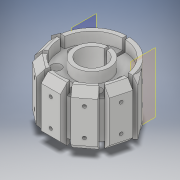
# Autodesk Inventor part: Sensor_Mount
Saved by Autodesk Inventor 2019.3 (Build 233278000, 278)
## iProperties
Created: 2019-04-10
Part Number: Sensor_Mount
Material: Типовые
Document SubType Name: Modeling
Designer: Andrew
Density: 1 g/cm^3
Appearance: По умолчанию
Author: Andrew
## iProperties of the stored document Sensor_Mount_3DПЕЧАТЬ.ipt
Created: 2019-04-10
Part Number: Sensor_Mount_3DПЕЧАТЬ
Material: Типовые
Document SubType Name: Modeling
Designer: Andrew
Density: 1 g/cm^3
Appearance: По умолчанию
Author: Andrew
Autodesk Inventor part; units mm, degrees
ref_plane "YZ Plane" through (0, 0, 0) normal (1, 0, 0) x (0, 1, 0)
ref_plane "XZ Plane" through (0, 0, 0) normal (0, 1, 0) x (-1, 0, 0)
ref_plane "XY Plane" through (0, 0, 0) normal (0, 0, 1) x (1, 0, 0)
sketch "Эскиз3" plane through (0, 0, 0) normal (0, 1, 0) x (-1, 0, 0)
  line L0 (-27.0893, -3.0942) -> (-31.566, -1.8947) construction
  line L1 (-31.566, -1.8947) -> (-26.3896, 17.4238) construction
  line L2 (-26.3896, 17.4238) -> (-21.9129, 16.2243) construction
  line L3 (-21.9129, 16.2243) -> (-27.0893, -3.0942) construction
  line L4 (-22.6894, 13.3265) -> (-27.166, 14.5261)
  line L5 (-27.166, 14.5261) -> (-30.7895, 1.0031)
  line L6 (-30.7895, 1.0031) -> (-26.3128, -0.1964)
  line L7 (-26.3128, -0.1964) -> (-22.6894, 13.3265)
  line L8 (-28.9778, 7.7646) -> (0, 0) construction
  line L9 (-23.375, 14.0361) -> (-26.1964, 17.713) construction
  line L10 (-26.1964, 17.713) -> (-10.3293, 29.8882) construction
  line L11 (-10.3293, 29.8882) -> (-7.508, 26.2114) construction
  line L12 (-7.508, 26.2114) -> (-23.375, 14.0361) construction
  line L13 (-9.888, 24.3851) -> (-12.7094, 28.0619)
  line L14 (-12.7094, 28.0619) -> (-23.8163, 19.5393)
  line L15 (-23.8163, 19.5393) -> (-20.995, 15.8624)
  line L16 (-20.995, 15.8624) -> (-9.888, 24.3851)
  line L17 (-18.2628, 23.8006) -> (0, 0) construction
  line L18 (-10, 25.3654) -> (-10, 30) construction
  line L19 (-10, 30) -> (10, 30) construction
  line L20 (10, 30) -> (10, 25.3654) construction
  line L21 (10, 25.3654) -> (-10, 25.3654) construction
  line L22 (7, 25.3654) -> (7, 30)
  line L23 (7, 30) -> (-7, 30)
  line L24 (-7, 30) -> (-7, 25.3654)
  line L25 (-7, 25.3654) -> (7, 25.3654)
  line L26 (0, 30) -> (0, 0) construction
  line L27 (7.508, 26.2114) -> (10.3293, 29.8882) construction
  line L28 (10.3293, 29.8882) -> (26.1964, 17.713) construction
  line L29 (26.1964, 17.713) -> (23.375, 14.0361) construction
  line L30 (23.375, 14.0361) -> (7.508, 26.2114) construction
  line L31 (20.995, 15.8624) -> (23.8163, 19.5393)
  line L32 (23.8163, 19.5393) -> (12.7094, 28.0619)
  line L33 (12.7094, 28.0619) -> (9.888, 24.3851)
  line L34 (9.888, 24.3851) -> (20.995, 15.8624)
  line L35 (18.2628, 23.8006) -> (0, 0) construction
  line L36 (21.9129, 16.2243) -> (26.3896, 17.4238) construction
  line L37 (26.3896, 17.4238) -> (31.566, -1.8947) construction
  line L38 (31.566, -1.8947) -> (27.0893, -3.0942) construction
  line L39 (27.0893, -3.0942) -> (21.9129, 16.2243) construction
  line L40 (26.3128, -0.1964) -> (30.7895, 1.0031)
  line L41 (30.7895, 1.0031) -> (27.166, 14.5261)
  line L42 (27.166, 14.5261) -> (22.6894, 13.3265)
  line L43 (22.6894, 13.3265) -> (26.3128, -0.1964)
  line L44 (28.9778, 7.7646) -> (0, 0) construction
  arc A0 (1, -26.2946) -> (-1, -26.2946) centre (0, 0) ccw
  arc A1 (1, -9.8494) -> (-1, -9.8494) centre (0, 0) ccw
  line L45 (-1, -9.8494) -> (-1, -26.2946)
  line L46 (1, -26.2946) -> (1, -9.8494)
  arc A2 (-1, -26.2946) -> (1, -26.2946) centre (0, 0) ccw construction
  arc A3 (-1, -9.8494) -> (1, -9.8494) centre (0, 0) ccw construction
  line L47 (31.566, -1.8947) -> (26.0982, -3.3598)
  line L48 (31.566, -1.8947) -> (22.2932, -13.9792)
  line L49 (-26.0982, -3.3598) -> (-31.566, -1.8947)
  line L50 (-31.566, -1.8947) -> (-22.2932, -13.9792)
  point P0 (0, 0)
  point P1 (0, 0)
  point P2 (0, 0)
  point P3 (0, 0)
  point P4 (0, 0)
  dimension "d8" = 20
  dimension "d9" = 3
  dimension "d10" = 3
  dimension "d11" = 30
  dimension "d14" = 150
  dimension "d16" = 19.8
  constraints: 102 end point, 13 point on circle, 11 point on line, 5 parallel, 4 centre point, 3 coincident, 3 perpendicular, 1 collinear, 1 midpoint, 80 other
  measures "d8" distance between parallel lines of L2 L0
  measures "d9" distance between parallel lines of L0 L6
  measures "d10" distance between parallel lines of L2 L4
  measures "d11" distance of L8.start L8.end
  measures "d16" diameter of A1
extrude "Выдавливание1" add sketch "Эскиз3" along normal blind 40
sketch "Эскиз5" plane through (0, 40, 0) normal (0, 1, 0) x (1, 0, 0)
  arc A0 (-1, 9.8494) -> (1, 9.8494) centre (0, 0) ccw construction
  circle A1 centre (0, 0) radius 12.9
  circle A2 centre (0, 0) radius 23.3136
  arc A3 (-22.6894, -13.3265) -> (-20.995, -15.8624) centre (0, 0) ccw projected
  arc A4 (20.995, -15.8624) -> (22.6894, -13.3265) centre (0, 0) ccw projected
  arc A5 (7, -25.3654) -> (9.888, -24.3851) centre (0, 0) ccw projected
  arc A6 (-9.888, -24.3851) -> (-7, -25.3654) centre (0, 0) ccw projected
  line L0 (-22.6894, -13.3265) -> (-20.1026, -11.8072)
  line L1 (-20.995, -15.8624) -> (-18.6013, -14.0539)
  line L2 (-26.3128, 0.1964) -> (-23.3128, 0.1964)
  line L3 (-26.0982, 3.3598) -> (-23.0702, 3.3598)
  line L4 (-9.888, -24.3851) -> (-8.7607, -21.6049)
  line L5 (-7, -25.3654) -> (-6.2019, -22.4735)
  line L6 (9.888, -24.3851) -> (8.7607, -21.6049)
  line L7 (7, -25.3654) -> (6.2019, -22.4735)
  line L8 (22.6894, -13.3265) -> (20.2775, -11.5042)
  line L9 (20.995, -15.8624) -> (18.6013, -14.0539)
  line L10 (26.3128, 0.1964) -> (23.3129, 0.174)
  line L11 (26.0982, 3.3598) -> (23.0735, 3.3372)
  arc A7 (22.2932, 13.9792) -> (1, 26.2946) centre (0, 0) ccw construction
  arc A8 (26.3128, 0.1964) -> (26.0982, 3.3598) centre (0, 0) ccw projected
  arc A9 (-26.0982, 3.3598) -> (-26.3128, 0.1964) centre (0, 0) ccw projected
  point P0 (0, 0)
  dimension "d24" = 3
  dimension "d26" = 3
  constraints: 24 end point, 3 parallel, 2 coincident, 1 centre point, 1 horizontal, 22 other
  measures "d24" radial gap between concentric circles of A1 A0
extrude "Выдавливание2" cut sketch "Эскиз5" against normal blind 8
sketch "Эскиз6" plane through (0, 32, 0) normal (0, 1, 0) x (1, 0, 0)
  line L0 (0, 0) -> (48.0015, 0) construction
  line L1 (0, 0) -> (17.8806, 4.7911) construction
  point P0 (14.6861, -11.269)
  point P1 (0, -18.5114)
  point P2 (-14.6861, -11.269)
  point P3 (-17.8806, 4.7911)
  dimension "d29" = 15
  dimension "d32" = 210
  constraints: 4 end point, 1 coincident, 1 horizontal, 5 other
  measures "d29" angle of L0 L1
sketch "Эскиз7" plane through (0, 0, 0) normal (0, -1, 0) x (1, 0, 0)
  line L0 (-1, -23.2921) -> (-1, -12.8612) projected
  arc A0 (-23.0702, -3.3598) -> (-1, -23.2921) centre (0, 0) ccw projected
  line L1 (-26.0982, -3.3598) -> (-23.0702, -3.3598) projected
  arc A1 (-26.3128, -0.1964) -> (-26.0982, -3.3598) centre (0, 0) ccw projected
  line L2 (-23.3128, -0.1964) -> (-26.3128, -0.1964) projected
  arc A2 (-20.1026, 11.8072) -> (-23.3128, -0.1964) centre (0, 0) ccw projected
  line L3 (-22.6894, 13.3265) -> (-20.1026, 11.8072) projected
  arc A3 (-20.995, 15.8624) -> (-22.6894, 13.3265) centre (0, 0) ccw projected
  line L4 (-18.6013, 14.0539) -> (-20.995, 15.8624) projected
  arc A4 (-8.7607, 21.6049) -> (-18.6013, 14.0539) centre (0, 0) ccw projected
  line L5 (-9.888, 24.3851) -> (-8.7607, 21.6049) projected
  arc A5 (-7, 25.3654) -> (-9.888, 24.3851) centre (0, 0) ccw projected
  line L6 (-6.2019, 22.4735) -> (-7, 25.3654) projected
  arc A6 (6.2019, 22.4735) -> (-6.2019, 22.4735) centre (0, 0) ccw projected
  line L7 (7, 25.3654) -> (6.2019, 22.4735) projected
  arc A7 (9.888, 24.3851) -> (7, 25.3654) centre (0, 0) ccw projected
  line L8 (8.7607, 21.6049) -> (9.888, 24.3851) projected
  arc A8 (18.6013, 14.0539) -> (8.7607, 21.6049) centre (0, 0) ccw projected
  line L9 (20.995, 15.8624) -> (18.6013, 14.0539) projected
  arc A9 (22.6894, 13.3265) -> (20.995, 15.8624) centre (0, 0) ccw projected
  line L10 (20.2775, 11.5042) -> (22.6894, 13.3265) projected
  arc A10 (23.3129, -0.174) -> (20.2775, 11.5042) centre (0, 0) ccw projected
  line L11 (26.3128, -0.1964) -> (23.3129, -0.174) projected
  arc A11 (26.0982, -3.3598) -> (26.3128, -0.1964) centre (0, 0) ccw projected
  line L12 (23.0735, -3.3372) -> (26.0982, -3.3598) projected
  arc A12 (1, -23.2921) -> (23.0735, -3.3372) centre (0, 0) ccw projected
  line L13 (1, -12.8612) -> (1, -23.2921) projected
  arc A13 (1, -12.8612) -> (-1, -12.8612) centre (0, 0) ccw projected
  point P0 (0, 0)
extrude "Выдавливание3" cut sketch "Эскиз7" against normal blind 5
hole "Отверстие1" at (17.8806, 32, -4.7911) at (-17.8806, 32, -4.7911) at (-14.6861, 32, 11.269) at (0, 32, 18.5114) at (14.6861, 32, 11.269) direction (0, -1, 0) diameter 7 end through all
ref_plane "РабПлоскость1" through (-24, 0, -9.8494) normal (-1, 0, 0) x (0, 0, 1)
sketch "Эскиз9" plane through (-24, 0, -9.8494) normal (-1, 0, 0) x (0, 0, 1)
  line L0 (-4.1298, 40) -> (-16.4452, 40) projected
  point P0 (9.8494, 0)
  point P1 (-11.0652, 25)
  point P2 (-11.0652, 10)
  dimension "d44" = 15
  dimension "d45" = 15
  constraints: 1 vertical alignment
  measures "d44" distance from line of L0 point (-11.065, 25)
  measures "d45" distance of point (-11.065, 10) point (-11.065, 25)
hole "Отверстие2" at (-24, 25, -20.9145) at (-24, 10, -20.9145) direction (1, 0, 0) diameter 3.2 end through all counterbore diameter 6 counterbore depth 15
ref_plane "РабПлоскость2" through (19, 0, -26.2946) normal (1, 0, 0) x (0, 0, -1)
sketch "Эскиз10" plane through (19, 0, -26.2946) normal (1, 0, 0) x (0, 0, -1)
  circle A0 centre (-5.38, 25) radius 3
  circle A1 centre (-5.38, 25) radius 1.6 projected
  circle A2 centre (-5.38, 10) radius 3
  circle A3 centre (-5.38, 10) radius 1.6 projected
  point P0 (-26.2946, 0)
  dimension "d54" = 6
  dimension "d55" = 6
  constraints: 2 centre point, 2 horizontal alignment, 4 other
  measures "d54" diameter of A0
  measures "d55" diameter of A2
extrude "Выдавливание4" cut sketch "Эскиз10" against normal blind 8
sketch "Эскиз11" plane through (-27.166, 0, 14.5261) normal (-0.9659258, 0, 0.258819) x (0.258819, 0, 0.9659258)
  line L0 (0, 0) -> (-14, 0) projected
  line L1 (0, 0) -> (0, 40) projected
  line L2 (-14, 40) -> (0, 40) projected
  line L3 (-14, 0) -> (-14, 40) projected
  line L4 (-14, 20) -> (0, 20)
  point P0 (-7, 0)
  point P1 (-7, 10)
  point P2 (-7, 30)
  dimension "d58" = 20
  constraints: 2 end point, 2 midpoint, 1 symmetric about line
  measures "d58" diameter of point (-7, 10) L4
sketch "Эскиз12" plane through (-12.7094, 0, 28.0619) normal (-0.6087614, 0, 0.7933533) x (0.7933533, 0, 0.6087614)
  line L0 (0, 0) -> (-14, 0)
  line L1 (0, 0) -> (0, 40)
  line L2 (-14, 40) -> (0, 40)
  line L3 (-14, 0) -> (-14, 40)
  line L4 (-14, 20) -> (0, 20)
  point P0 (-7, 0)
  point P1 (-7, 0)
  point P2 (-7, 10)
  point P3 (-7, 30)
  dimension "d59" = 20
  constraints: 10 end point, 2 midpoint, 1 symmetric about line
  measures "d59" diameter of point (-7, 10) L4
hole "Отверстие3" at (-28.9778, 30, 7.7646) at (-28.9778, 10, 7.7646) direction (0.9659258, 0, -0.258819) diameter 2.4 depth 8 tip angle 118
hole "Отверстие4" at (-18.2628, 10, 23.8006) at (-18.2628, 30, 23.8006) direction (0.6087614, 0, -0.7933533) diameter 2.4 depth 8 tip angle 118
sketch "Эскиз14" plane through (-7, 0, 30) normal (0, 0, 1) x (1, 0, 0)
  line L0 (14, 0) -> (0, 0)
  line L1 (14, 0) -> (14, 40)
  line L2 (0, 40) -> (14, 40)
  line L3 (0, 0) -> (0, 40)
  line L4 (0, 20) -> (14, 20)
  point P0 (7, 0)
  point P1 (7, 0)
  point P2 (7, 0)
  point P3 (7, 10)
  point P4 (7, 30)
  dimension "d74" = 20
  constraints: 10 end point, 2 midpoint, 1 symmetric about line
  measures "d74" diameter of point (7, 10) L4
hole "Отверстие5" at (0, 10, 30) at (0, 30, 30) direction (0, 0, -1) diameter 2.4 depth 8 tip angle 118
sketch "Эскиз15" plane through (23.8163, 0, 19.5393) normal (0.6087614, 0, 0.7933533) x (0.7933533, 0, -0.6087614)
  line L0 (0, 0) -> (-14, 0)
  line L1 (0, 0) -> (0, 40)
  line L2 (-14, 40) -> (0, 40)
  line L3 (-14, 0) -> (-14, 40)
  line L4 (-14, 20) -> (0, 20)
  point P0 (-7, 0)
  point P1 (-7, 0)
  point P2 (-7, 10)
  point P3 (-7, 30)
  dimension "d82" = 20
  constraints: 10 end point, 2 midpoint, 1 symmetric about line
  measures "d82" diameter of point (-7, 10) L4
hole "Отверстие6" at (18.2628, 10, 23.8006) at (18.2628, 30, 23.8006) direction (-0.6087614, 0, -0.7933533) diameter 2.4 depth 8 tip angle 118
sketch "Эскиз16" plane through (30.7895, 0, 1.0031) normal (0.9659258, 0, 0.258819) x (0.258819, 0, -0.9659258)
  line L0 (0, 0) -> (-14, 0)
  line L1 (0, 0) -> (0, 40)
  line L2 (-14, 40) -> (0, 40)
  line L3 (-14, 0) -> (-14, 40)
  line L4 (-14, 20) -> (0, 20)
  point P0 (-7, 0)
  point P1 (-7, 0)
  point P2 (-7, 10)
  point P3 (-7, 30)
  dimension "d90" = 20
  constraints: 10 end point, 2 midpoint, 1 symmetric about line
  measures "d90" diameter of point (-7, 10) L4
hole "Отверстие7" at (28.9778, 10, 7.7646) at (28.9778, 30, 7.7646) direction (-0.9659258, 0, -0.258819) diameter 2.4 depth 8 tip angle 118
chamfer "Фаска2" distance 5 angle 45 10 edges at (-28.9778, 40, 7.7646) (-18.2628, 40, 23.8006) (0, 40, 30) (18.2628, 40, 23.8006) (28.9778, 40, 7.7646) (-28.9778, 0, 7.7646) (-18.2628, 0, 23.8006) (0, 0, 30) (18.2628, 0, 23.8006) (28.9778, 0, 7.7646)
chamfer "Фаска3" distance 3 angle 45 4 edges at (-26.9296, 40, -7.9369) (26.9296, 40, -7.9369) (-26.9296, 0, -7.9369) (26.9296, 0, -7.9369)
